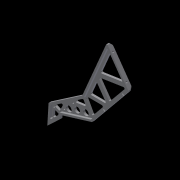
# Autodesk Inventor part: Stock
Saved by Autodesk Inventor 2020.4 (Build 244396010, 396A)
## iProperties
Created: 2022-09-10
Part Number: Stock
Material: Generic
Document SubType Name: Modeling
Designer: Val
Density: 1 g/cm^3
Appearance: Default
Author: Val
Autodesk Inventor part; units mm, degrees
ref_plane "YZ Plane" through (0, 0, 0) normal (1, 0, 0) x (0, 1, 0)
ref_plane "XZ Plane" through (0, 0, 0) normal (0, 1, 0) x (-1, 0, 0)
ref_plane "XY Plane" through (0, 0, 0) normal (0, 0, 1) x (1, 0, 0)
sketch "Base" plane through (0, 0, 0) normal (0, 0, 1) x (1, 0, 0)
  line L0 (-48.3105, 274.7583) -> (-44.1704, 343.479)
  line L1 (-4.8622, 327.8071) -> (101.9965, 360.4139)
  line L2 (101.9965, 360.4139) -> (225.313, 510.5952)
  line L3 (225.313, 510.5952) -> (151.6386, 615.2993)
  line L4 (151.6386, 615.2993) -> (68.9003, 421.0435)
  line L5 (-44.1704, 343.479) -> (68.9003, 421.0435)
  line L6 (-5.6371, 314.9459) -> (-48.3105, 274.7583)
  line L7 (-5.6371, 314.9459) -> (-4.8622, 327.8071)
  point P0 (0, 0)
  constraints: 16 end point, 1 parallel
extrude "BaseFeature" add sketch "Base" along normal mid plane 28.575
sketch "Holes" plane through (0, 0, -14.2875) normal (0, 0, -1) x (-1, 0, 0)
  line L0 (-101.9965, 360.4139) -> (4.8622, 327.8071) construction
  line L1 (4.8622, 327.8071) -> (5.6371, 314.9459) construction
  line L2 (5.6371, 314.9459) -> (48.3105, 274.7583) construction
  line L3 (48.3105, 274.7583) -> (44.1704, 343.479) construction
  line L4 (44.1704, 343.479) -> (-68.9003, 421.0435) construction
  line L5 (-68.9003, 421.0435) -> (-151.6386, 615.2993) construction
  line L6 (-151.6386, 615.2993) -> (-225.313, 510.5952) construction
  line L7 (-225.313, 510.5952) -> (-101.9965, 360.4139) construction
  line L8 (14.1512, 331.5105) -> (32.9904, 339.0216)
  line L9 (4.8622, 327.8071) -> (-101.9965, 360.4139) projected
  line L10 (14.0908, 320.721) -> (36.8124, 299.323)
  line L11 (36.8124, 299.323) -> (35.0206, 329.0656)
  line L12 (-82.59, 375.0942) -> (-65.4275, 406.5345) construction
  line L13 (-69.6311, 419.7046) -> (-73.7165, 412.2206) construction
  line L14 (-95.7962, 371.7724) -> (-134.875, 419.3647)
  line L15 (-134.875, 419.3647) -> (-83.5162, 419.6323)
  line L16 (-88.3079, 430.8823) -> (-144.0937, 430.5917)
  line L17 (-88.3079, 430.8823) -> (-109.2658, 480.0881)
  line L18 (-109.2658, 480.0881) -> (-144.0937, 430.5917)
  line L19 (-208.929, 509.5515) -> (-153.3124, 441.8187)
  line L20 (-153.3124, 441.8187) -> (-115.7207, 495.2429)
  line L21 (-225.313, 510.5952) -> (-151.6386, 615.2993) projected
  line L22 (-115.7207, 495.2429) -> (-208.929, 509.5515)
  line L23 (-122.1755, 510.3978) -> (-199.9341, 522.3346)
  line L24 (-199.9341, 522.3346) -> (-154.6629, 586.6729)
  line L25 (-154.6629, 586.6729) -> (-122.1755, 510.3978)
  line L26 (-208.929, 509.5515) -> (-199.9341, 522.3346) construction
  line L27 (-109.2658, 480.0881) -> (-122.1755, 510.3978) construction
  line L28 (-134.875, 419.3647) -> (-153.3124, 441.8187) construction
  line L29 (-101.9965, 360.4139) -> (-68.9003, 421.0435) construction
  line L30 (-68.9003, 421.0435) -> (44.1704, 343.479) projected
  line L31 (4.8622, 327.8071) -> (44.1704, 343.479) construction
  line L32 (14.0908, 320.721) -> (35.0206, 329.0656)
  line L33 (32.9904, 339.0216) -> (-65.4275, 406.5345) construction
  circle A0 centre (-74.2295, 370.5304) radius 9.525
  circle A1 centre (-44.93, 363.779) radius 9.525
  circle A2 centre (-16.8526, 353.0225) radius 9.525
  arc A3 (-16.8526, 353.0225) -> (-74.2295, 370.5304) centre (-107.9414, 157.2786) ccw construction
  line L34 (14.1512, 331.5105) -> (-1.9993, 363.0239)
  line L35 (32.9904, 339.0216) -> (-1.9993, 363.0239)
  line L36 (-65.4275, 406.5345) -> (-75.1933, 388.6443)
  line L37 (-29.5446, 381.9195) -> (-65.4275, 406.5345)
  line L38 (-75.1933, 388.6443) -> (-29.5446, 381.9195)
  line L39 (-73.7165, 412.2206) -> (-83.5162, 419.6323)
  line L40 (-73.7165, 412.2206) -> (-95.7962, 371.7724)
  line L41 (-83.5162, 419.6323) -> (-69.6311, 419.7046) construction
  line L42 (-65.4275, 406.5345) -> (-73.7165, 412.2206) construction
  line L43 (-83.5162, 419.6323) -> (-88.3079, 430.8823) construction
  point P0 (0, 0)
  dimension "d25" = 19.05
  dimension "d3" = 14
  dimension "d4" = 14
  dimension "d8" = 14
  dimension "d9" = 14
  dimension "d11" = 11.2749
  dimension "d13" = 10
  dimension "d14" = 10
  dimension "d19" = 10
  dimension "d21" = 10
  dimension "d24" = 10
  dimension "d27" = 17.78
  dimension "d28" = 17.78
  dimension "d29" = 215.9
  dimension "d30" = 17.78
  dimension "d31" = 17.78
  dimension "d32" = 30.0673
  dimension "d33" = 30.0673
  dimension "d34" = 10
  dimension "d35" = 12
  constraints: 66 end point, 17 parallel, 10 collinear, 4 point on line, 3 centre point, 3 point on circle, 2 midpoint, 1 coincident, 1 equal radius, 5 other
  measures "d3" distance between parallel lines of L5 L17
  measures "d4" distance between parallel lines of L6 L24
  measures "d8" distance between parallel lines of L23 L22
  measures "d9" distance between parallel lines of L20 L18
  measures "d11" distance between parallel lines of L16 L15
  measures "d13" distance between parallel lines of L3 L11
  measures "d14" distance between parallel lines of L2 L10
  measures "d19" distance between parallel lines of L13 L12
  measures "d21" distance between parallel lines of L8 L32
  measures "d24" distance between parallel lines of L4 L33
  measures "d27" distance from line of L0 A3.end
  measures "d28" distance from line of L0 A2.centre
  measures "d29" radius of A3
  measures "d30" distance from line of L38 A3.end
  measures "d31" distance from line of A2.centre L34
  measures "d32" distance of A1.centre A3.end
  measures "d33" distance of A2.centre A1.centre
  measures "d34" distance of L0.end L8.start
  measures "d35" distance between parallel lines of L7 L19
extrude "HolesFeature" cut sketch "Holes" against normal through all
chamfer "ChamfersFeature" distance 6.35 angle 45 12 edges at (-5.2497, 321.3765, -14.2875) (48.5671, 344.1105, -14.2875) (163.6548, 435.5045, -14.2875) (110.2695, 518.1714, -14.2875) (12.365, 382.2612, -14.2875) (-46.2404, 309.1187, -14.2875) (-5.2497, 321.3765, 14.2875) (48.5671, 344.1105, 14.2875) (163.6548, 435.5045, 14.2875) (110.2695, 518.1714, 14.2875) (12.365, 382.2612, 14.2875) (-46.2404, 309.1187, 14.2875)
fillet "FilletsFEature" radius 3.175 38 edges at (95.7962, 371.7724, 0) (134.875, 419.3647, 0) (29.5446, 381.9195, 0) (75.1933, 388.6443, 0) (65.4275, 406.5345, 0) (-32.9904, 339.0216, 0) (-14.1512, 331.5105, 0) (1.9993, 363.0239, 0) (-14.0908, 320.721, 0) (-36.8124, 299.323, 0) (-35.0206, 329.0656, 0) (109.2658, 480.0881, 0) (144.0937, 430.5917, 0) (88.3079, 430.8823, 0) (153.3124, 441.8187, 0) (115.7207, 495.2429, 0) (208.929, 509.5515, 0) (122.1755, 510.3978, 0) (199.9341, 522.3346, 0) (154.6629, 586.6729, 0) (-4.8622, 327.8071, 0) (-5.6371, 314.9459, 0) (101.9965, 360.4139, 0) (225.313, 510.5952, 0) (68.9003, 421.0435, 0) (-44.1704, 343.479, 0) (151.6386, 615.2993, 0) (73.7165, 412.2206, 0) (83.5162, 419.6323, 0) (100.1518, 363.1705, -11.1125) (223.4172, 513.2895, -11.1125) (223.4172, 513.2895, 11.1125) (100.1518, 363.1705, 11.1125) (153.7884, 612.2441, -11.1125) (153.7884, 612.2441, 11.1125) (-41.0945, 341.7388, -11.1125) (-41.0945, 341.7388, 11.1125) (71.459, 418.9484, -11.1125)
split "HalfSplitFeature" plane through (0, 0, 0) removes the side toward (0, 0, 1)
sketch "Hollow" plane through (69.2627, 421.8943, 0) normal (0, 0, 1) x (0.9200244, -0.391861, 0)
  line L0 (108.133, 140.439) -> (54.4774, -42.8152) projected
  arc A0 (108.133, 140.439) -> (106.7589, 144.0296) centre (105.086, 141.3312) ccw projected
  line L1 (4.848, 207.2116) -> (106.7589, 144.0296) projected
  arc A1 (4.848, 207.2116) -> (0, 204.5131) centre (3.175, 204.5131) ccw projected
  line L2 (0, 0) -> (0, 204.5131) projected
  line L3 (-72.7998, -115.2847) -> (-0.4966, -1.705) projected
  arc A2 (-0.4966, -1.705) -> (0, 0) centre (-3.175, 0) ccw projected
  arc A3 (53.4728, -44.3539) -> (54.4774, -42.8152) centre (51.4303, -41.9231) ccw projected
  line L4 (53.4728, -44.3539) -> (-29.6387, -114.1901) projected
  arc A4 (-72.7998, -115.2847) -> (-73.1121, -118.056) centre (-70.1215, -116.9897) ccw projected
  line L5 (-50.5133, -181.4411) -> (-73.1121, -118.056) projected
  arc A5 (-29.6387, -114.1901) -> (-30.5868, -117.6871) centre (-27.5962, -116.6209) ccw projected
  line L6 (-30.5868, -117.6871) -> (-27.4236, -126.5593) projected
  arc A6 (-27.5058, -128.8991) -> (-27.4236, -126.5593) centre (-30.4142, -127.6255) ccw projected
  line L7 (-27.5058, -128.8991) -> (-50.5133, -181.4411) projected
  line L8 (48.653, -40.1098) -> (101.3602, 139.9054)
  line L9 (101.3602, 139.9054) -> (6.35, 198.809)
  line L10 (6.35, 198.809) -> (6.35, 0)
  arc A7 (4.8601, -5.115) -> (6.35, 0) centre (-3.175, 0) ccw
  line L11 (4.8601, -5.115) -> (-66.6096, -117.3854)
  line L12 (-66.6096, -117.3854) -> (-51.6967, -159.2132)
  line L13 (-49.9085, -164.229) -> (-33.8278, -127.5056) construction
  line L14 (-33.8278, -127.5056) -> (-35.616, -122.4898) construction
  arc A8 (-33.7238, -109.3285) -> (-36.568, -119.8196) centre (-27.5962, -116.6209) ccw
  line L15 (-33.7238, -109.3285) -> (48.653, -40.1098)
  line L16 (-35.616, -122.4898) -> (-51.6967, -159.2132)
  line L17 (-46.35, -147.0029) -> (-39.0398, -130.3086) projected
  line L18 (-35.616, -122.4898) -> (-36.568, -119.8196)
  line L19 (-51.6967, -159.2132) -> (-49.9085, -164.229) construction
  point P0 (101.6006, -415.2944)
  dimension "d55" = 6.35
  dimension "d56" = 6.35
  dimension "d57" = 6.35
  dimension "d58" = 6.35
  constraints: 22 end point, 4 point on circle, 2 centre point, 1 collinear, 1 tangent, 5 other
  measures "d55" distance between parallel lines of L0 L8
  measures "d56" distance between parallel lines of L4 L15
  measures "d57" distance between parallel lines of L18 L6
  measures "d58" distance between parallel lines of L5 L12
extrude "HollowFeature" cut sketch "Hollow" against normal blind 7 contours L15 A8 L18 L16 L12 L11 A7 L10 L9 L8
fillet "HollowFilletsFeature" radius 3.175 6 edges at (-40.689, 295.6722, -3.5) (-38.0186, 339.9986, -3.5) (-11.5039, 323.1572, -3.5) (98.3072, 365.9272, -3.5) (217.34, 510.8916, -3.5) (153.0104, 602.3152, -3.5)
sketch "HalfJoinHoles" plane through (0, 0, -14.2875) normal (0, 0, -1) x (-1, 0, 0)
  circle A0 centre (-209.0662, 515.9302) radius 3
  circle A1 centre (-155.9016, 592.6885) radius 3
  circle A2 centre (-31.1388, 377.5134) radius 3
  circle A3 centre (33.1348, 334.1009) radius 3
  circle A4 centre (-1.5991, 344.7591) radius 3
  point P0 (0, 0)
  dimension "d42" = 6
  dimension "d43" = 6
  dimension "d44" = 6
  dimension "d45" = 6
  dimension "d46" = 6
  constraints: 5 centre point
  measures "d42" diameter of A0
  measures "d43" diameter of A1
  measures "d44" diameter of A2
  measures "d45" diameter of A3
  measures "d46" diameter of A4
extrude "HalfJoinHolesFeature" cut sketch "HalfJoinHoles" against normal through all
sketch "MountHoles" plane through (-6.5539, 314.0825, -8.8007) normal (0.6855851, -0.7279925, 0) x (0.7279925, 0.6855851, 0)
  line L0 (0, 8.8007) -> (-57.3586, 8.8007) construction
  line L1 (-57.3586, 0.8632) -> (-57.3586, 8.8007) construction
  line L2 (-48.0946, -5.4868) -> (-57.3586, 0.8632) construction
  line L3 (-8.0047, -5.4868) -> (-48.0946, -5.4868) construction
  line L4 (0, 0) -> (-8.0047, -5.4868) construction
  line L5 (0, 8.8007) -> (0, 0) construction
  circle A0 centre (-39.5786, 2.4507) radius 3.175
  line L6 (-39.5786, 2.4507) -> (-12.7, 2.4507) construction
  circle A1 centre (-12.7, 2.4507) radius 3.175
  point P0 (-210.5591, 8.8007)
  dimension "d49" = 6.35
  dimension "d50" = 6.35
  dimension "d51" = 17.78
  dimension "d52" = 12.7
  constraints: 2 centre point, 2 end point, 1 coincident, 1 equal radius, 1 horizontal
  measures "d49" diameter of A0
  measures "d50" distance between parallel lines of L0 L6
  measures "d51" distance from line of L1 L6.start
  measures "d52" distance from line of L5 L6.end
extrude "MountHolesFeature" cut sketch "MountHoles" against normal blind 12.7
sketch "EndMountHoles" plane through (223.9231, 512.5705, 0) normal (0.8178294, 0.5754607, 0) x (0, 0, -1)
  line L0 (0, 119.9075) -> (0, 0) projected
  line L1 (6.6224, 0) -> (0, 0) projected
  line L2 (14.2875, 7.9536) -> (6.6224, 0) projected
  line L3 (14.2875, 110.8887) -> (14.2875, 7.9536) projected
  line L4 (6.6224, 119.9075) -> (14.2875, 110.8887) projected
  line L5 (0, 119.9075) -> (6.6224, 119.9075) projected
  circle A0 centre (6, 20.32) radius 3
  line L6 (6, 20.32) -> (6, 99.5875) construction
  circle A1 centre (6, 99.5875) radius 3
  point P0 (0, -290.3362)
  dimension "d60" = 6
  dimension "d61" = 6
  dimension "d62" = 6
  dimension "d63" = 20.32
  dimension "d64" = 20.32
  constraints: 2 centre point, 2 end point, 1 coincident, 1 vertical
  measures "d60" diameter of A0
  measures "d61" distance from line of L0 L6.start
  measures "d62" diameter of A1
  measures "d63" distance from line of L1 L6.start
  measures "d64" distance from line of L5 L6.end
extrude "EndMountHolesFeature" cut sketch "EndMountHoles" against normal up to surface (6.35 mm away) contours A0 | A1
sketch "Sketch8" plane through (102.6056, 361.1557, 0) normal (0.772844, -0.634596, 0) x (0, 0, -1)
  circle A0 centre (0, 167.5317) radius 2.5 projected
  circle A1 centre (0, 67.5317) radius 2.5 projected
  point P0 (0, -344.2301)
hole "Hole1" at (145.461, 413.3472, 0) at (208.9206, 490.6316, 0) direction (-0.772844, 0.634596, 0) diameter 5 depth 12
equation "\"d9\" = d8"
equation "\"d13\" = d2"
equation "\"d14\" = d2"
equation "\"d19\" = d2"
equation "\"d21\" = d2"
equation "\"d24\" = d2"
equation "\"d2\" = 10"
body "Solid1"
